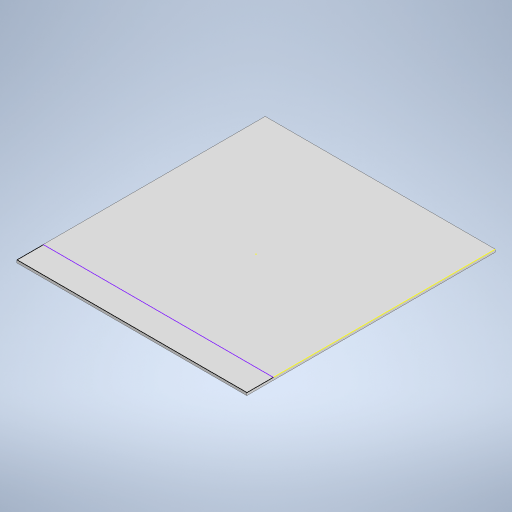
# Autodesk Inventor part: Bottom
Saved by Autodesk Inventor 2023 (Build 270158000, 158)
## iProperties
Created: 2024-05-13
Part Number: Bottom
Material: Generic
Document SubType Name: Modeling
Designer: noname
Density: 1 g/cm^3
Appearance: Default
Author: noname
Autodesk Inventor part; units mm, degrees
ref_plane "YZ Plane" through (0, 0, 0) normal (1, 0, 0) x (0, 1, 0)
ref_plane "XZ Plane" through (0, 0, 0) normal (0, 1, 0) x (-1, 0, 0)
ref_plane "XY Plane" through (0, 0, 0) normal (0, 0, 1) x (1, 0, 0)
sketch "Sketch1" plane through (0, 0, 0) normal (0, 1, 0) x (-1, 0, 0)
  line L0 (50, 54) -> (-50, 54)
  line L1 (-50, 54) -> (-50, -54)
  line L2 (-50, -54) -> (50, -54)
  line L3 (50, -54) -> (50, 54)
  line L4 (50, 54) -> (-50, -54) construction
  line L5 (-50, 54) -> (50, -54) construction
  point P0 (0, 0)
  dimension "d0" = 108
  dimension "d1" = 100
  constraints: 12 end point, 2 midpoint, 2 parallel, 1 horizontal, 1 perpendicular
  measures "d0" distance between parallel lines of L0 L2
  measures "d1" distance between parallel lines of L3 L1
extrude "Extrusion1" add sketch "Sketch1" along normal blind 1.2
sketch "Sketch2" plane through (0, 1.2, 0) normal (0, 1, 0) x (1, 0, 0)
  line L0 (-50, -54) -> (50, -54) projected
  line L1 (50, -54) -> (50, 54) projected
  line L2 (-50, -54) -> (50, -54)
  line L3 (50, -54) -> (50, -42.5315)
  line L4 (50, -42.5315) -> (-50, -42.5315)
  line L5 (-50, -42.5315) -> (-50, -54)
  point P0 (0, 0)
  constraints: 8 end point, 2 parallel, 1 horizontal, 1 perpendicular, 1 point on line
body "Solid1"
